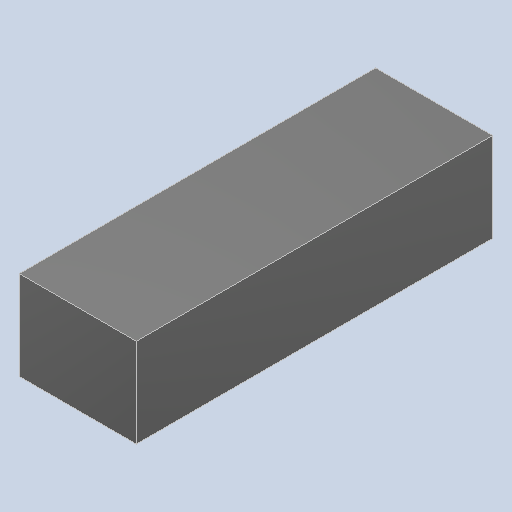
# Autodesk Inventor part: batterie
Saved by Autodesk Inventor 2024 (Build 280153000, 153)
## iProperties
Created: 2022-11-09
Part Number: batterie
Material: Thermoplastic Resin
Document SubType Name: Modeling
Designer: Thomas
Density: 1.28 g/cm^3
Appearance: Smooth - Black
Mass: 288.512 g
Surface Area: 259 cm^2
Volume: 225.4 cm^3
Author: Thomas
Autodesk Inventor part; units mm, degrees
ref_plane "YZ Plane" through (0, 0, 0) normal (1, 0, 0) x (0, 1, 0)
ref_plane "XZ Plane" through (0, 0, 0) normal (0, 1, 0) x (-1, 0, 0)
ref_plane "XY Plane" through (0, 0, 0) normal (0, 0, 1) x (1, 0, 0)
sketch "Sketch1" plane through (0, 0, 0) normal (0, 0, 1) x (1, 0, 0)
  line L0 (-23, -17.5) -> (23, -17.5)
  line L1 (23, -17.5) -> (23, 17.5)
  line L2 (23, 17.5) -> (-23, 17.5)
  line L3 (-23, 17.5) -> (-23, -17.5)
  line L4 (-23, -17.5) -> (23, 17.5) construction
  line L5 (23, -17.5) -> (-23, 17.5) construction
  point P0 (0, 0)
  dimension "d0" = 35
  dimension "d1" = 46
  constraints: 12 end point, 2 midpoint, 2 parallel, 1 horizontal, 1 perpendicular
  measures "d0" distance of L0.end L1.end
  measures "d1" distance of L1.end L2.end
extrude "Extrusion1" add sketch "Sketch1" along normal blind 140
body "Solid1"
